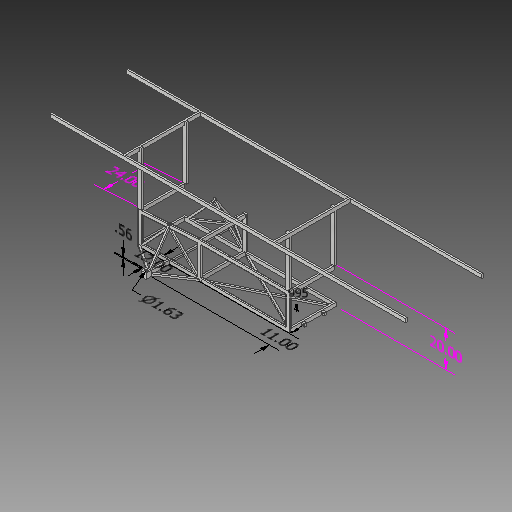
# Autodesk Inventor part: finalDoneskies
Saved by Autodesk Inventor 2018 (Build 220112000, 112)
## iProperties
Created: 2018-01-31
Part Number: finalDoneskies
Material: Generic
Document SubType Name: Modeling
Designer: rochee19
Density: 1 g/cm^3
Appearance: Default
Author: rochee19
Autodesk Inventor part; units mm, degrees
ref_plane "YZ Plane" through (0, 0, 0) normal (1, 0, 0) x (0, 1, 0)
ref_plane "XZ Plane" through (0, 0, 0) normal (0, 1, 0) x (-1, 0, 0)
ref_plane "XY Plane" through (0, 0, 0) normal (0, 0, 1) x (1, 0, 0)
sketch "Sketch1" plane through (0, 0, 0) normal (0, 0, 1) x (1, 0, 0)
  line L0 (0, 0) -> (2133.6, 0)
  line L1 (2133.6, 0) -> (2133.6, -50.8)
  line L2 (2133.6, -50.8) -> (0, -50.8)
  line L3 (0, -50.8) -> (0, 0)
  line L4 (2133.6, 0) -> (2082.8, 0)
  line L5 (2082.8, 0) -> (2082.8, 457.2)
  line L6 (2082.8, 457.2) -> (2133.6, 457.2)
  line L7 (2133.6, 457.2) -> (2133.6, 0)
  line L8 (0, 0) -> (50.8, 0)
  line L9 (50.8, 0) -> (50.8, 406.4)
  line L10 (50.8, 406.4) -> (0, 406.4)
  line L11 (0, 406.4) -> (0, 0)
  line L12 (50.8, 203.2) -> (838.2, 203.2)
  line L13 (838.2, 0) -> (889, 0)
  line L14 (889, 0) -> (889, 457.2)
  line L15 (889, 457.2) -> (838.2, 457.2)
  line L16 (838.2, 457.2) -> (838.2, 0)
  dimension "d0" = 2133.6
  dimension "d1" = 50.8
  dimension "d2" = 50.8
  dimension "d3" = 457.2
  dimension "d4" = 50.8
  dimension "d5" = 406.4
  dimension "d6" = 787.4
  dimension "d7" = 50.8
  dimension "d8" = 457.2
  constraints: 34 end point, 8 parallel, 5 horizontal, 4 perpendicular, 1 midpoint, 1 point on line
  measures "d0" distance of L1.end L2.end
  measures "d1" distance of L0.end L1.end
  measures "d2" distance of L5.end L6.end
  measures "d3" distance of L4.end L5.end
  measures "d4" distance of L10.end L9.end
  measures "d5" distance of L9.end L8.end
  measures "d6" distance of L12.start L12.end
  measures "d7" distance of L15.end L14.end
  measures "d8" distance of L14.end L13.end
extrude "Extrusion1" add sketch "Sketch1" along normal blind 25.4 contours L11 L10 L9 L0 | L16 L15 L14 L0 | L0 L5 L6 L7
sketch "Sketch2" plane through (0, 0, 25.4) normal (0, 0, 1) x (1, 0, 0)
  line L0 (0, 0) -> (50.8, 0) projected
  line L1 (0, 0) -> (2133.6, 0)
  line L2 (2133.6, 0) -> (2133.6, -50.8)
  line L3 (2133.6, -50.8) -> (0, -50.8)
  line L4 (0, -50.8) -> (0, 0)
  dimension "d11" = 2133.6
  dimension "d12" = 50.8
  constraints: 8 end point, 2 parallel, 1 horizontal, 1 perpendicular
  measures "d11" distance of L2.end L3.end
  measures "d12" distance of L1.end L2.end
extrude "Extrusion2" add sketch "Sketch2" against normal blind 25.4
sketch "Sketch3" plane through (0, 0, 25.4) normal (0, 0, 1) x (1, 0, 0)
  line L0 (838.2, 457.2) -> (838.2, 0) projected
  line L1 (50.8, 406.4) -> (0, 406.4) projected
  line L2 (838.2, 457.2) -> (25.4, 406.4)
  line L3 (25.4, 406.4) -> (28.5688, 355.6989)
  line L4 (28.5688, 355.6989) -> (841.3688, 406.4989)
  line L5 (841.3688, 406.4989) -> (838.2, 457.2)
  line L6 (889, 0) -> (889, 457.2) projected
  line L7 (2082.8, 457.2) -> (2082.8, 0) projected
  line L8 (889, 457.2) -> (2082.8, 457.2)
  line L9 (2082.8, 457.2) -> (2082.8, 406.4)
  line L10 (2082.8, 406.4) -> (889, 406.4)
  line L11 (889, 406.4) -> (889, 457.2)
  point P0 (0, 0)
  dimension "d15" = 50.8
  constraints: 16 end point, 4 parallel, 3 perpendicular, 1 midpoint
  measures "d15" distance of L3.end L2.end
extrude "Extrusion3" add sketch "Sketch3" against normal blind 25.4
shell "Shell1" thickness 2.54 removed faces 0
sketch "Sketch5" plane through (0, 0, 0) normal (0, 0, -1) x (-1, 0, 0)
  line L0 (-2133.6, -50.8) -> (0, -50.8) projected
  line L1 (0, -50.8) -> (-25.4, -50.8)
  line L2 (-25.4, -50.8) -> (-25.4, 0)
  line L3 (-25.4, 0) -> (0, 0)
  line L4 (0, 0) -> (0, -50.8)
  line L5 (-2133.6, 457.2) -> (-2133.6, -50.8) projected
  line L6 (-2133.6, -50.8) -> (-2108.2, -50.8)
  line L7 (-2108.2, -50.8) -> (-2108.2, 0)
  line L8 (-2108.2, 0) -> (-2133.6, 0)
  line L9 (-2133.6, 0) -> (-2133.6, -50.8)
  line L10 (-2082.8, 406.4) -> (-889, 0) projected
  line L11 (-889, 0) -> (-889, -50.8)
  line L12 (-838.2, 406.3009) -> (-838.2, 0) projected
  line L13 (-838.2, 0) -> (-838.2, -50.8)
  line L14 (-838.2, -25.4) -> (-889, -25.4)
  line L15 (-876.3, -50.8) -> (-850.9, -50.8)
  line L16 (-850.9, -50.8) -> (-850.9, 0)
  line L17 (-850.9, 0) -> (-876.3, 0)
  line L18 (-876.3, 0) -> (-876.3, -50.8)
  line L19 (-876.3, -50.8) -> (-850.9, 0) construction
  line L20 (-850.9, -50.8) -> (-876.3, 0) construction
  line L21 (-838.2, -25.4) -> (-25.4, -25.4)
  line L22 (-431.8, -25.4) -> (-431.8, 0)
  line L23 (-48.26, -2.54) -> (-840.74, -2.54) projected
  line L24 (-431.8, 0) -> (-431.8, -50.8)
  line L25 (-50.8, 0) -> (-838.2, 0) projected
  line L26 (-444.5, -50.8) -> (-419.1, -50.8)
  line L27 (-419.1, -50.8) -> (-419.1, 0)
  line L28 (-419.1, 0) -> (-444.5, 0)
  line L29 (-444.5, 0) -> (-444.5, -50.8)
  line L30 (-444.5, -50.8) -> (-419.1, 0) construction
  line L31 (-419.1, -50.8) -> (-444.5, 0) construction
  point P0 (-863.6, -25.4)
  point P1 (-788.4519, -2.54)
  point P2 (-776.7012, 0)
  dimension "d23" = 25.4
  dimension "d24" = 50.8
  dimension "d25" = 25.4
  dimension "d26" = 25.4
  dimension "d27" = 50.8
  dimension "d28" = 25.4
  constraints: 52 end point, 9 midpoint, 8 parallel, 7 perpendicular, 6 point on line, 4 horizontal
  measures "d23" distance of L2.end L3.end
  measures "d24" distance of L1.end L2.end
  measures "d25" distance of L8.end L7.end
  measures "d26" distance of L17.end L16.end
  measures "d27" distance of L16.end L15.end
  measures "d28" distance of L28.end L27.end
extrude "Extrusion5" add sketch "Sketch5" along normal blind 609.6 contours L5 L8 L7 L0 | L18 L14 L16 L0 | L18 L17 L16 L14 | L29 L21 L24 L0 | L24 L21 L27 L0 | L29 L23 L22 L21 | L22 L23 L27 L21 | L29 L25 L22 L23 | L2 L3 L4 L0 | L22 L25 L27 L23
sketch "Sketch6" plane through (0, 0, -609.6) normal (0, 0, -1) x (-1, 0, 0)
  line L0 (-2133.6, 457.2) -> (-2133.6, -50.8) projected
  line L1 (-2133.6, -50.8) -> (0, -50.8)
  line L2 (0, -50.8) -> (0, 0)
  line L3 (0, 0) -> (-2133.6, 0)
  line L4 (-2133.6, 0) -> (-2133.6, -50.8)
  constraints: 8 end point, 2 parallel, 1 horizontal, 1 perpendicular
extrude "Extrusion6" add sketch "Sketch6" along normal blind 25.4
sketch "Sketch7" plane through (0, 0, -635) normal (0, 0, -1) x (-1, 0, 0)
  line L0 (-889, 0) -> (-838.2, 0)
  line L1 (-838.2, 0) -> (-838.2, 457.2)
  line L2 (-838.2, 457.2) -> (-889, 457.2)
  line L3 (-889, 457.2) -> (-889, 0)
  line L4 (0, 406.4) -> (0, -50.8) projected
  line L5 (0, 406.4) -> (-50.8, 406.4)
  line L6 (-50.8, 406.4) -> (-50.8, 0)
  line L7 (-50.8, 0) -> (0, 0)
  line L8 (0, 0) -> (0, 406.4)
  line L9 (-2133.6, 0) -> (-2133.6, -50.8) projected
  line L10 (-2133.6, 0) -> (-2082.8, 0)
  line L11 (-2082.8, 0) -> (-2082.8, 457.2)
  line L12 (-2082.8, 457.2) -> (-2133.6, 457.2)
  line L13 (-2133.6, 457.2) -> (-2133.6, 0)
  line L14 (-2082.8, 406.4) -> (-889, 406.4)
  line L15 (-889, 406.4) -> (-889, 457.2)
  line L16 (-889, 457.2) -> (-2082.8, 457.2)
  line L17 (-2082.8, 457.2) -> (-2082.8, 406.4)
  line L18 (-25.4, 406.4) -> (0, 406.4) projected
  line L19 (-838.2, 457.2) -> (-25.4, 406.4)
  line L20 (-25.4, 406.4) -> (-28.5688, 355.6989)
  line L21 (-28.5688, 355.6989) -> (-841.3688, 406.4989)
  line L22 (-841.3688, 406.4989) -> (-838.2, 457.2)
  line L23 (-838.2, 406.3009) -> (-50.8, 357.0884) projected
  line L24 (-50.8, 357.0884) -> (-838.2, 0) projected
  line L25 (-50.8, 357.0884) -> (-838.2, 0)
  line L26 (-838.2, 0) -> (-827.7094, -23.1324)
  line L27 (-827.7094, -23.1324) -> (-40.3094, 333.956)
  line L28 (-40.3094, 333.956) -> (-50.8, 357.0884)
  line L29 (-2082.8, 406.4) -> (-889, 406.4) projected
  dimension "d33" = 50.8
  dimension "d34" = 457.2
  dimension "d35" = 50.8
  dimension "d36" = 457.2
  dimension "d37" = 50.8
  dimension "d38" = 25.4
  constraints: 48 end point, 13 equal length, 6 perpendicular, 4 horizontal
  measures "d33" distance of L2.end L1.end
  measures "d34" distance of L1.end L0.end
  measures "d35" distance of L12.end L11.end
  measures "d36" distance of L11.end L10.end
  measures "d37" distance of L18.start L20.end
  measures "d38" distance of L26.end L0.end
extrude "Extrusion7" [suppressed]
sketch "Sketch8" plane through (0, 0, -635) normal (0, 0, -1) x (-1, 0, 0)
  line L0 (0, 0) -> (-2133.6, 0) projected
  line L1 (-889, 0) -> (-838.2, 0)
  line L2 (-838.2, 0) -> (-838.2, 457.2)
  line L3 (-838.2, 457.2) -> (-889, 457.2)
  line L4 (-889, 457.2) -> (-889, 0)
  dimension "d42" = 50.8
  dimension "d43" = 457.2
  constraints: 8 end point, 2 parallel, 1 horizontal, 1 perpendicular
  measures "d42" distance of L3.end L2.end
  measures "d43" distance of L2.end L1.end
extrude "Extrusion8" add sketch "Sketch8" against normal blind 25.4
sketch "Sketch9" plane through (0, 0, 0) normal (0, 0, -1) x (-1, 0, 0)
  line L0 (0, 406.4) -> (0, 0) projected
  line L1 (0, 406.4) -> (-25.4, 406.4)
  line L2 (-25.4, 406.4) -> (-25.4, 355.6)
  line L3 (-25.4, 355.6) -> (0, 355.6)
  line L4 (0, 355.6) -> (0, 406.4)
  dimension "d46" = 25.4
  dimension "d47" = 50.8
  constraints: 8 end point, 2 parallel, 1 horizontal, 1 perpendicular
  measures "d46" distance of L3.end L2.end
  measures "d47" distance of L2.end L1.end
sketch "Sketch10" plane through (0, 0, -635) normal (0, 0, -1) x (-1, 0, 0)
  line L0 (-889, 457.2) -> (-889, 0) projected
  line L1 (-50.8, 357.0884) -> (-838.2, 406.3009) projected
  line L2 (-889, 406.4) -> (-838.2, 406.3009)
  line L3 (-838.2, 406.3009) -> (-863.6, 406.3504)
  line L4 (-889, 457.2) -> (-838.2, 457.2) projected
  line L5 (-863.6, 457.2) -> (-863.6, 406.3504)
  line L6 (-876.3, 406.3752) -> (-850.9, 406.3752)
  line L7 (-850.9, 406.3752) -> (-850.9, 457.1752)
  line L8 (-850.9, 457.1752) -> (-876.3, 457.1752)
  line L9 (-876.3, 457.1752) -> (-876.3, 406.3752)
  line L10 (-876.3, 406.3752) -> (-850.9, 457.1752) construction
  line L11 (-850.9, 406.3752) -> (-876.3, 457.1752) construction
  point P0 (0, 0)
  point P1 (-2133.6, 457.2)
  point P2 (-863.6, 431.7752)
  dimension "d48" = 25.4
  dimension "d49" = 50.8
  constraints: 18 end point, 5 midpoint, 2 parallel, 2 perpendicular, 1 horizontal
  measures "d48" distance of L8.end L7.end
  measures "d49" distance of L7.end L6.end
extrude "Extrusion9" add sketch "Sketch10" against normal blind 635 contours L9 L8 L5 L6 | L8 L7 L6 L5
extrude "Extrusion10" add sketch "Sketch9" along normal blind 609.6
sketch "Sketch11" plane through (0, 0, 0) normal (0, 0, -1) x (-1, 0, 0)
  line L0 (-889, 457.2) -> (-838.2, 457.2) projected
  line L1 (-2133.6, 457.2) -> (-2108.2, 457.2)
  line L2 (-2108.2, 457.2) -> (-2108.2, 406.4)
  line L3 (-2108.2, 406.4) -> (-2133.6, 406.4)
  line L4 (-2133.6, 406.4) -> (-2133.6, 457.2)
  point P0 (0, 0)
  dimension "d54" = 25.4
  dimension "d55" = 50.8
  constraints: 8 end point, 2 parallel, 1 horizontal, 1 perpendicular
  measures "d54" distance of L2.end L3.end
  measures "d55" distance of L1.end L2.end
extrude "Extrusion11" add sketch "Sketch11" along normal blind 609.6
sketch "Sketch12" plane through (2133.6, -50.8, 25.4) normal (1, 0, 0) x (0, 0, -1)
  line L0 (635, 0) -> (635, 50.8) projected
  line L1 (635, 50.8) -> (635, 0)
  line L2 (635, 25.4) -> (0, 25.4)
  line L3 (0, 508) -> (0, 0) projected
  line L4 (25.4, 50.8) -> (0, 50.8) projected
  line L5 (25.4, 50.8) -> (25.4, 0)
  line L6 (22.86, 2.54) -> (22.86, 505.46) projected
  line L7 (25.4, 50.8) -> (25.4, 0) projected
  line L8 (25.4, 25.4) -> (635, 25.4)
  line L9 (330.2, 25.4) -> (330.2, 50.8)
  line L10 (25.4, 50.8) -> (635, 50.8) projected
  line L11 (330.2, 25.4) -> (209.55, 25.4)
  line L12 (209.55, 25.4) -> (450.85, 25.4)
  line L13 (450.85, 25.4) -> (482.6, 25.4)
  line L14 (450.85, 6.35) -> (450.85, 44.45)
  line L15 (450.85, 44.45) -> (482.6, 44.45)
  line L16 (482.6, 44.45) -> (482.6, 6.35)
  line L17 (482.6, 6.35) -> (450.85, 6.35)
  line L18 (450.85, 6.35) -> (482.6, 44.45) construction
  line L19 (450.85, 44.45) -> (482.6, 6.35) construction
  line L20 (209.55, 25.4) -> (177.8, 25.4)
  line L21 (177.8, 25.4) -> (209.55, 25.4)
  line L22 (177.8, 6.35) -> (177.8, 44.45)
  line L23 (177.8, 44.45) -> (209.55, 44.45)
  line L24 (209.55, 44.45) -> (209.55, 6.35)
  line L25 (209.55, 6.35) -> (177.8, 6.35)
  line L26 (177.8, 6.35) -> (209.55, 44.45) construction
  line L27 (177.8, 44.45) -> (209.55, 6.35) construction
  point P0 (466.725, 25.4)
  point P1 (193.675, 25.4)
  dimension "d58" = 120.65
  dimension "d59" = 241.3
  dimension "d60" = 31.75
  dimension "d61" = 38.1
  dimension "d62" = 31.75
  dimension "d63" = 38.1
  constraints: 44 end point, 10 midpoint, 5 parallel, 5 point on line, 4 perpendicular, 2 collinear, 1 horizontal, 1 vertical
  measures "d58" distance of L9.start L11.end
  measures "d59" distance of L11.end L12.end
  measures "d60" distance of L12.end L13.end
  measures "d61" distance of L14.start L14.end
  measures "d62" distance of L11.end L20.end
  measures "d63" distance of L22.start L22.end
extrude "Extrusion12" add sketch "Sketch12" along normal blind 38.1 contours L16 L17 L14 L2 | L2 L14 L15 L16 | L24 L25 L22 L2 | L2 L22 L23 L24
sketch "Sketch13" plane through (2133.6, -44.45, -152.4) normal (0, 0, 1) x (1, 0, 0)
  line L0 (0, 38.1) -> (38.1, 38.1) projected
  line L1 (19.05, 38.1) -> (19.05, 0)
  line L2 (0, 0) -> (38.1, 0) projected
  circle A0 centre (19.05, 19.05) radius 8.128
  point P0 (-2133.6, 44.45)
  dimension "d66" = 16.256
  constraints: 3 midpoint, 2 end point, 1 centre point
  measures "d66" diameter of A0
extrude "Extrusion13" cut sketch "Sketch13" against normal blind 38.1
sketch "Sketch14" plane through (2133.6, -44.45, -457.2) normal (0, 0, -1) x (-1, 0, 0)
  line L0 (0, 38.1) -> (-38.1, 38.1) projected
  line L1 (-19.05, 38.1) -> (-19.05, 0)
  line L2 (0, 0) -> (-38.1, 0) projected
  circle A0 centre (-19.05, 19.05) radius 8.128
  point P0 (2133.6, 44.45)
  constraints: 3 midpoint, 2 end point, 1 centre point
extrude "Extrusion14" cut sketch "Sketch14" against normal blind 38.1
sketch "Sketch23" plane through (0, 0, 25.4) normal (0, 0, 1) x (1, 0, 0)
  line L0 (50.8, 0) -> (50.8, 357.0884) projected
  line L1 (50.8, 0) -> (50.8, -50.8)
  line L2 (2133.6, -50.8) -> (0, -50.8) projected
  line L3 (50.8, 357.0884) -> (838.2, 0) projected
  line L4 (838.2, 0) -> (838.2, -50.8)
  line L5 (838.2, -50.8) -> (838.2, -25.4)
  line L6 (838.2, -25.4) -> (50.8, -25.4)
  line L7 (419.1, 0) -> (419.1, -50.8) projected
  line L8 (419.1, -25.4) -> (419.1, 0)
  line L9 (419.1, 0) -> (419.1, -50.8)
  line L10 (419.1, 0) -> (444.5, 0)
  line L11 (50.8, 0) -> (2082.8, 0) projected
  line L12 (444.5, -50.8) -> (444.5, 0) projected
  line L13 (444.5, -50.8) -> (444.5, 0)
  line L14 (444.5, 0) -> (444.5, -25.4)
  line L15 (419.1, -50.8) -> (444.5, -50.8)
  line L16 (444.5, -50.8) -> (444.5, 0)
  line L17 (444.5, 0) -> (419.1, 0)
  line L18 (419.1, 0) -> (419.1, -50.8)
  line L19 (419.1, -50.8) -> (444.5, 0) construction
  line L20 (444.5, -50.8) -> (419.1, 0) construction
  point P0 (0, 0)
  point P1 (50.8, 329.1985)
  point P2 (776.7012, 0)
  point P3 (431.8, -25.4)
  constraints: 30 end point, 6 midpoint, 3 collinear, 3 point on line, 2 parallel, 2 vertical, 1 horizontal, 1 perpendicular
extrude "Extrusion20" add sketch "Sketch23" along normal blind 279.4 contours L10 L12 L6 L7 | L6 L12 L2 L7
sketch "Sketch24" plane through (0, 0, -635) normal (0, 0, -1) x (-1, 0, 0)
  line L0 (-444.5, 0) -> (-444.5, -50.8)
  line L1 (-444.5, -50.8) -> (-419.1, -50.8)
  line L2 (-419.1, -50.8) -> (-419.1, 0)
  line L3 (-419.1, 0) -> (-444.5, 0)
  line L4 (0, 0) -> (-838.2, 0) projected
  point P0 (-50.8, 0)
  point P1 (-776.7012, 0)
  constraints: 8 end point, 2 perpendicular, 1 collinear, 1 vertical
extrude "Extrusion21" add sketch "Sketch24" along normal blind 279.4
sketch "Sketch25" plane through (2133.6, -50.8, -635) normal (0, -1, 0) x (1, 0, 0)
  line L0 (-2133.6, 660.4) -> (-2133.6, 0) projected
  line L1 (-1714.5, 660.4) -> (-1714.5, 939.8) projected
  line L2 (-2133.6, 660.4) -> (-1714.5, 939.8)
  line L3 (-1714.5, 939.8) -> (-1700.4106, 918.6659)
  line L4 (-1700.4106, 918.6659) -> (-2119.5106, 639.2659)
  line L5 (-2119.5106, 639.2659) -> (-2133.6, 660.4)
  line L6 (-1714.5, 939.8) -> (-2133.6, 660.4)
  line L7 (-1714.5, 939.8) -> (-1689.1, 939.8) projected
  line L8 (-1689.1, 939.8) -> (-1269.9857, 660.4)
  line L9 (0, 660.4) -> (-1295.4, 660.4) projected
  line L10 (-1269.9857, 660.4) -> (-1286.2971, 635.9321)
  line L11 (-1286.2971, 635.9321) -> (-1705.4114, 915.3321)
  line L12 (-1705.4114, 915.3321) -> (-1689.1, 939.8)
  point P0 (-2133.6, 635)
  dimension "d102" = 25.4
  dimension "d103" = 503.7074
  dimension "d104" = 503.7074
  constraints: 18 end point, 3 equal length, 3 perpendicular, 2 point on line
  measures "d102" distance of L1.end L3.end
  measures "d103" distance of L7.end L8.end
  measures "d104" distance of L10.end L11.end
extrude "Extrusion22" add sketch "Sketch25" against normal blind 25.4
sketch "Sketch26" plane through (2133.6, -50.8, -635) normal (0, -1, 0) x (1, 0, 0)
  line L0 (-1714.5, 0) -> (-1714.5, -279.4) projected
  line L1 (-2133.6, 25.4) -> (-2133.6, 660.4) projected
  line L2 (-1714.5, -279.4) -> (-2133.6, 0)
  line L3 (-2133.6, 0) -> (-2119.5106, 21.1341)
  line L4 (-2119.5106, 21.1341) -> (-1700.4106, -258.2659)
  line L5 (-1700.4106, -258.2659) -> (-1714.5, -279.4)
  line L6 (-1689.1, 0) -> (-1689.1, -279.4) projected
  line L7 (-1689.1, -279.4) -> (-1266.2023, -5.7603)
  line L8 (-1266.2023, -5.7603) -> (-1280.0009, 15.5648)
  line L9 (-1280.0009, 15.5648) -> (-1702.8986, -258.0749)
  line L10 (-1702.8986, -258.0749) -> (-1689.1, -279.4)
  point P0 (-2133.6, 635)
  dimension "d107" = 25.4
  dimension "d108" = 503.7074
  dimension "d109" = 25.4
  constraints: 16 end point, 4 parallel, 2 perpendicular
  measures "d107" distance of L2.end L3.end
  measures "d108" distance of L6.end L7.end
  measures "d109" distance of L8.end L7.end
extrude "Extrusion23" add sketch "Sketch26" against normal blind 25.4
sketch "Sketch28" plane through (419.1, -50.8, -635) normal (-1, 0, 0) x (0, 0, 1)
  line L0 (879.0384, 50.8) -> (617.9284, 448.692) projected
  line L1 (42.4716, 448.692) -> (-218.6384, 50.8) projected
  line L2 (617.9284, 448.692) -> (42.4716, 448.692)
  line L3 (42.4716, 448.692) -> (42.4716, 499.492)
  line L4 (42.4716, 499.492) -> (617.9284, 499.492)
  line L5 (617.9284, 499.492) -> (617.9284, 448.692)
  line L6 (-279.4, 50.8) -> (0, 476.5632) projected
  line L7 (42.4716, 499.492) -> (0, 476.5632)
  line L8 (0, 476.5632) -> (24.1328, 431.8614)
  line L9 (24.1328, 431.8614) -> (66.6043, 454.7902)
  line L10 (66.6043, 454.7902) -> (42.4716, 499.492)
  line L11 (660.4, 50.8) -> (660.4, 0) projected
  line L12 (617.9284, 499.492) -> (660.4, 476.5632)
  line L13 (660.4, 476.5632) -> (636.2672, 431.8614)
  line L14 (636.2672, 431.8614) -> (593.7957, 454.7902)
  line L15 (593.7957, 454.7902) -> (617.9284, 499.492)
  point P0 (635, 50.8)
  point P1 (660.4, 432.4946)
  dimension "d116" = 50.8
  dimension "d117" = 50.8
  dimension "d118" = 50.8
  constraints: 24 end point, 6 parallel, 3 perpendicular, 1 horizontal
  measures "d116" distance of L1.start L3.end
  measures "d117" distance of L8.end L6.end
  measures "d118" distance of L12.end L13.end
extrude "Extrusion25" add sketch "Sketch28" against normal blind 25.4
sketch "Sketch29" plane through (2133.6, -50.8, -635) normal (0, -1, 0) x (1, 0, 0)
  line L0 (-1257.3, 25.4) -> (-1257.3, 635) projected
  line L1 (-25.4, 635) -> (-1295.4, 635) projected
  line L2 (-1257.3, 25.4) -> (-25.4, 635)
  line L3 (-25.4, 635) -> (-14.1347, 612.2348)
  line L4 (-14.1347, 612.2348) -> (-1246.0347, 2.6348)
  line L5 (-1246.0347, 2.6348) -> (-1257.3, 25.4)
  line L6 (-1257.3, 635) -> (-1282.7, 635) projected
  line L7 (-1257.3, 635) -> (-25.4, 25.4)
  line L8 (-25.4, 25.4) -> (-14.1347, 48.1652)
  line L9 (-14.1347, 48.1652) -> (-1246.0347, 657.7652)
  line L10 (-1246.0347, 657.7652) -> (-1257.3, 635)
  point P0 (-2133.6, 635)
  dimension "d121" = 25.4
  dimension "d122" = 25.4
  constraints: 16 end point, 4 parallel, 2 perpendicular
  measures "d121" distance of L1.start L3.end
  measures "d122" distance of L8.end L7.end
extrude "Extrusion26" add sketch "Sketch29" against normal blind 25.4 contours L2 L7 L4 L5 | L10 L9 L1 | L1 L9 L2 L7 | L2 L9 L4 L7 | L2 L3 L4 L9 | L4 L9 L8 L7
extrude "Extrusion28" [suppressed]
sketch "Sketch33" plane through (0, -12.7, -596.9) normal (0, 0, 1) x (1, 0, 0)
  line L0 (-152.4, 0) -> (-152.4, 12.7) projected
  line L1 (0, 12.7) -> (-152.4, 12.7) projected
  line L2 (-152.4, 0) -> (-139.7, 0)
  line L3 (-139.7, 0) -> (-139.7, 12.7)
  line L4 (-139.7, 12.7) -> (-152.4, 12.7)
  line L5 (-152.4, 12.7) -> (-152.4, 0)
  line L6 (-152.4, 368.3) -> (-152.4, 381) projected
  line L7 (0, 368.3) -> (-152.4, 368.3) projected
  line L8 (-152.4, 381) -> (-139.7, 381)
  line L9 (-139.7, 381) -> (-139.7, 368.3)
  line L10 (-139.7, 368.3) -> (-152.4, 368.3)
  line L11 (-152.4, 368.3) -> (-152.4, 381)
  dimension "d139" = 12.7
  dimension "d140" = 12.7
  constraints: 16 end point, 4 parallel, 2 horizontal, 2 perpendicular, 2 point on line
  measures "d139" distance of L4.end L3.end
  measures "d140" distance of L9.end L10.end
extrude "Extrusion29" [suppressed]
sketch "Sketch51" plane through (444.5, -50.8, -635) normal (1, 0, 0) x (0, 0, -1)
  line L0 (-939.8, 25.4) -> (-939.8, 50.8) projected
  line L1 (-617.9284, 499.492) -> (-647.7476, 483.3937) projected
  line L2 (-939.8, 50.8) -> (-647.7476, 483.3937)
  line L3 (-647.7476, 483.3937) -> (-626.696, 469.1814)
  line L4 (-626.696, 469.1814) -> (-918.7484, 36.5877)
  line L5 (-918.7484, 36.5877) -> (-939.8, 50.8)
  line L6 (279.4, 50.8) -> (279.4, 25.4) projected
  line L7 (0, 476.5632) -> (-42.4716, 499.492) projected
  line L8 (279.4, 50.8) -> (-12.6524, 483.3937)
  line L9 (-12.6524, 483.3937) -> (-33.704, 469.1814)
  line L10 (-33.704, 469.1814) -> (258.3484, 36.5877)
  line L11 (258.3484, 36.5877) -> (279.4, 50.8)
  point P0 (-635, 50.8)
  dimension "d223" = 25.4
  dimension "d224" = 25.4
  constraints: 16 end point, 4 parallel, 2 perpendicular
  measures "d223" distance of L1.end L3.end
  measures "d224" distance of L9.end L8.end
extrude "Extrusion44" add sketch "Sketch51" against normal blind 25.4
sketch "Sketch74" plane through (0, 0, -635) normal (0, 0, -1) x (-1, 0, 0)
  line L0 (-2133.6, 457.2) -> (-2133.6, 406.4) projected
  line L1 (-2133.6, 406.4) -> (-2133.6, 457.2)
  line L2 (-2133.6, 457.2) -> (-2146.3, 457.2) projected
  line L3 (-2133.6, 457.2) -> (-2082.8, 457.2)
  line L4 (-2082.8, 457.2) -> (-2082.8, 1168.4)
  line L5 (-2082.8, 1168.4) -> (-2133.6, 1168.4)
  line L6 (-2133.6, 1168.4) -> (-2133.6, 457.2)
  line L7 (0, -25.4) -> (0, 0) projected
  line L8 (0, 406.4) -> (-50.8, 406.4)
  line L9 (-50.8, 406.4) -> (-50.8, 1168.4)
  line L10 (-50.8, 1168.4) -> (0, 1168.4)
  line L11 (0, 1168.4) -> (0, 406.4)
  dimension "d275" = 50.8
  dimension "d276" = 711.2
  dimension "d277" = 50.8
  constraints: 18 end point, 5 equal length, 2 horizontal, 2 perpendicular, 1 point on line
  measures "d275" distance of L5.end L4.end
  measures "d276" distance of L4.end L3.end
  measures "d277" distance of L9.end L10.end
extrude "Extrusion62" add sketch "Sketch74" against normal blind 25.4
sketch "Sketch75" plane through (0, 0, 25.4) normal (0, 0, 1) x (1, 0, 0)
  line L0 (0, 406.4) -> (0, -25.4) projected
  line L1 (0, 406.4) -> (50.8, 406.4)
  line L2 (50.8, 406.4) -> (50.8, 1168.4)
  line L3 (50.8, 1168.4) -> (0, 1168.4)
  line L4 (0, 1168.4) -> (0, 406.4)
  line L5 (838.2, 457.2) -> (889, 457.2) projected
  line L6 (2133.6, 1168.4) -> (2082.8, 1168.4) projected
  line L7 (2133.6, 457.2) -> (2082.8, 457.2)
  line L8 (2082.8, 457.2) -> (2082.8, 1168.4)
  line L9 (2082.8, 1168.4) -> (2133.6, 1168.4)
  line L10 (2133.6, 1168.4) -> (2133.6, 457.2)
  point P0 (0, 0)
  point P1 (2139.95, 457.2)
  constraints: 16 end point, 4 parallel, 2 horizontal, 2 perpendicular
extrude "Extrusion63" add sketch "Sketch75" against normal blind 25.4
sketch "Sketch79" plane through (2133.6, -50.8, 25.4) normal (1, 0, 0) x (0, 0, -1)
  line L0 (25.4, 407.8884) -> (25.4, 50.8) projected
  point P0 (635, 1193.8)
extrude "Extrusion66" [suppressed]
sketch "Sketch80" plane through (0, 0, 25.4) normal (0, 0, 1) x (1, 0, 0)
  line L0 (48.26, -2.54) -> (48.26, 359.4746) projected
  line L1 (444.5, 397.892) -> (419.1, 397.892) projected
  line L2 (48.26, -2.54) -> (419.1, 397.892)
  line L3 (419.1, 397.892) -> (437.7359, 380.6333)
  line L4 (437.7359, 380.6333) -> (66.8959, -19.7987)
  line L5 (66.8959, -19.7987) -> (48.26, -2.54)
  line L6 (838.2, 406.3009) -> (838.2, 0) projected
  line L7 (838.2, 0) -> (443.4121, 397.892)
  line L8 (443.4121, 397.892) -> (425.3814, 380.0019)
  line L9 (425.3814, 380.0019) -> (820.1693, -17.89)
  line L10 (820.1693, -17.89) -> (838.2, 0)
  point P0 (0, 0)
  dimension "d293" = 25.4
  dimension "d294" = 25.4
  constraints: 16 end point, 4 parallel, 2 perpendicular
  measures "d293" distance of L1.end L3.end
  measures "d294" distance of L8.end L7.end
extrude "Extrusion67" add sketch "Sketch80" against normal blind 25.4 contours L7 L10 L9 L4 L3 L8 | L3 L8 L9 L4 L5 L2 | L3 L4 L9 L8
sketch "Sketch81" plane through (0, 0, 25.4) normal (0, 0, 1) x (1, 0, 0)
  line L0 (2082.8, 406.4) -> (2082.8, 0) projected
  line L1 (889, 0) -> (2082.8, 0) projected
  point P0 (0, 0)
extrude "Extrusion68" [suppressed]
sketch "Sketch82" plane through (0, 0, -635) normal (0, 0, -1) x (-1, 0, 0)
  line L0 (-50.8, 357.0884) -> (-838.2, 0) projected
  line L1 (-50.8, 357.0884) -> (-838.2, 0)
  line L2 (-838.2, 0) -> (-827.7094, -23.1324)
  line L3 (-827.7094, -23.1324) -> (-40.3094, 333.956)
  line L4 (-40.3094, 333.956) -> (-50.8, 357.0884)
  point P0 (0, 0)
  dimension "d300" = 25.4
  constraints: 8 end point, 3 equal length, 1 perpendicular
  measures "d300" distance of L2.end L0.end
extrude "Extrusion69" cut sketch "Sketch82" against normal blind 25.4
sketch "Sketch83" plane through (0, 0, -635) normal (0, 0, -1) x (-1, 0, 0)
  line L0 (-458.6082, 382.5764) -> (-838.2, 0) projected
  line L1 (-444.5, 396.7955) -> (-456.2305, 384.9727) projected
  line L2 (-838.2, 0) -> (-444.5, 396.7955)
  line L3 (-838.2, 0) -> (-444.5, 396.7955)
  line L4 (-444.5, 396.7955) -> (-426.4693, 378.9054)
  line L5 (-426.4693, 378.9054) -> (-820.1693, -17.89)
  line L6 (-820.1693, -17.89) -> (-838.2, 0)
  line L7 (-50.8, 0.2027) -> (-50.8, 357.0884) projected
  line L8 (-50.8, 0.2027) -> (-422.297, 401.1418)
  line L9 (-422.297, 401.1418) -> (-440.9285, 383.8784)
  line L10 (-440.9285, 383.8784) -> (-69.4316, -17.0607)
  line L11 (-69.4316, -17.0607) -> (-50.8, 0.2027)
  point P0 (0, 0)
  dimension "d303" = 25.4
  constraints: 18 end point, 4 parallel, 2 perpendicular, 1 collinear
  measures "d303" distance of L9.end L8.end
extrude "Extrusion70" add sketch "Sketch83" against normal blind 25.4
sketch "Sketch84" plane through (0, 0, -635) normal (0, 0, -1) x (-1, 0, 0)
  line L0 (-838.2, 0) -> (-827.7094, -23.1324) projected
  line L1 (-827.7094, -23.1324) -> (-776.7012, 0) projected
  line L2 (-838.2, 0) -> (-776.7012, 0)
  line L3 (-776.7012, 0) -> (-776.7012, -23.1324)
  line L4 (-776.7012, -23.1324) -> (-838.2, -23.1324)
  line L5 (-838.2, -23.1324) -> (-838.2, 0)
  point P0 (0, 0)
  constraints: 8 end point, 2 parallel, 1 horizontal, 1 perpendicular
extrude "Extrusion71" add sketch "Sketch84" against normal blind 25.4 contours L2 L1 L0
sketch "Sketch85" plane through (0, 406.4, -609.6) normal (-1, 0, 0) x (0, 0, 1)
  line L0 (0, 762) -> (0, 50.8) projected
  line L1 (0, 762) -> (0, 749.3)
  line L2 (609.6, 762) -> (609.6, 736.6)
  line L3 (609.6, 50.8) -> (609.6, 762) projected
  line L4 (609.6, 736.6) -> (0, 736.6)
  line L5 (-245.491, 711.2) -> (855.091, 711.2)
  line L6 (855.091, 711.2) -> (855.091, 762)
  line L7 (855.091, 762) -> (-245.491, 762)
  line L8 (-245.491, 762) -> (-245.491, 711.2)
  line L9 (-245.491, 711.2) -> (855.091, 762) construction
  line L10 (855.091, 711.2) -> (-245.491, 762) construction
  point P0 (609.6, -406.4)
  point P1 (304.8, 736.6)
  dimension "d308" = 12.7
  dimension "d309" = 25.4
  dimension "d310" = 1100.582
  dimension "d311" = 50.8
  constraints: 18 end point, 3 midpoint, 3 point on line, 2 parallel, 2 perpendicular, 1 horizontal
  measures "d308" distance of L0.start L1.end
  measures "d309" distance of L2.start L2.end
  measures "d310" distance of L7.end L6.end
  measures "d311" distance of L6.end L5.end
extrude "Extrusion72" add sketch "Sketch85" against normal blind 25.4
sketch "Sketch86" plane through (2133.6, 457.2, 25.4) normal (1, 0, 0) x (0, 0, -1)
  line L0 (25.4, 711.2) -> (25.4, 0) projected
  line L1 (25.4, 711.2) -> (25.4, 685.8)
  line L2 (25.4, 685.8) -> (635, 685.8)
  line L3 (635, 711.2) -> (635, 0) projected
  line L4 (660.4, 660.4) -> (880.491, 660.4) projected
  line L5 (-220.091, 711.2) -> (880.491, 711.2)
  line L6 (880.491, 711.2) -> (880.491, 660.4)
  line L7 (880.491, 660.4) -> (-220.091, 660.4)
  line L8 (-220.091, 660.4) -> (-220.091, 711.2)
  line L9 (-220.091, 711.2) -> (880.491, 660.4) construction
  line L10 (880.491, 711.2) -> (-220.091, 660.4) construction
  point P0 (25.4, -457.2)
  point P1 (330.2, 685.8)
  dimension "d314" = 25.4
  constraints: 16 end point, 3 midpoint, 2 parallel, 2 perpendicular, 2 point on line, 1 horizontal
  measures "d314" distance of L0.start L1.end
extrude "Extrusion73" add sketch "Sketch86" against normal blind 25.4
sketch "Sketch87" plane through (0, 1117.6, 245.491) normal (0, 0, 1) x (1, 0, 0)
  line L0 (0, 50.8) -> (0, 0) projected
  line L1 (0, 50.8) -> (-1016, 50.8)
  line L2 (-1016, 50.8) -> (3987.8, 50.8)
  line L3 (3987.8, 50.8) -> (3987.8, 0)
  line L4 (3987.8, 0) -> (-1016, 0)
  line L5 (-1016, 0) -> (-1016, 50.8)
  point P0 (0, -1117.6)
  dimension "d317" = 1016
  dimension "d318" = 5003.8
  constraints: 10 end point, 2 horizontal, 2 parallel, 1 perpendicular
  measures "d317" distance of L0.start L1.end
  measures "d318" distance of L3.end L4.end
extrude "Extrusion74" add sketch "Sketch87" against normal blind 25.4
sketch "Sketch88" plane through (0, 1117.6, -855.091) normal (0, 0, -1) x (-1, 0, 0)
  line L0 (1016, 50.8) -> (0, 50.8) projected
  line L1 (-3987.8, 0) -> (-2133.6, 0) projected
  line L2 (1016, 50.8) -> (-3987.8, 50.8)
  line L3 (-3987.8, 50.8) -> (-3987.8, 0)
  line L4 (-3987.8, 0) -> (1016, 0)
  line L5 (1016, 0) -> (1016, 50.8)
  point P0 (0, -1117.6)
  constraints: 8 end point, 2 parallel, 1 horizontal, 1 perpendicular
extrude "Extrusion75" add sketch "Sketch88" against normal blind 25.4
sketch "Sketch95" plane through (0, 0, 304.8) normal (0, 0, 1) x (1, 0, 0)
  line L0 (443.8315, -50.8) -> (419.7685, -50.8) projected
  line L1 (431.8, -50.8) -> (466.725, -50.8)
  line L2 (431.8, -50.8) -> (396.875, -50.8)
  line L3 (419.1, -50.8) -> (444.5, -50.8) projected
  line L4 (396.875, -50.8) -> (396.875, 25.4)
  line L5 (396.875, 25.4) -> (466.725, 25.4)
  line L6 (466.725, 25.4) -> (466.725, -50.8)
  point P0 (0, 0)
  point P1 (71.5448, -50.8)
  dimension "d350" = 34.925
  dimension "d351" = 34.925
  dimension "d352" = 76.2
  constraints: 10 end point, 3 perpendicular, 1 collinear, 1 midpoint, 1 point on line
  measures "d350" distance of L1.start L1.end
  measures "d351" distance of L1.start L2.end
  measures "d352" distance of L2.end L4.end
extrude "Extrusion80" add sketch "Sketch95" along normal blind 69.85
sketch "Sketch96" plane through (396.875, 25.4, 304.8) normal (0, 1, 0) x (1, 0, 0)
  line L0 (69.85, 0) -> (0, 0) projected
  line L1 (34.925, 0) -> (34.925, -69.85)
  line L2 (69.85, -69.85) -> (0, -69.85) projected
  circle A0 centre (34.925, -34.925) radius 15.0812
  point P0 (-396.875, 304.8)
  dimension "d355" = 30.1625
  constraints: 3 midpoint, 2 end point, 1 centre point
  measures "d355" diameter of A0
extrude "Extrusion81" cut sketch "Sketch96" against normal blind 76.2
sketch "Sketch97" plane through (396.875, 25.4, 304.8) normal (0, 1, 0) x (1, 0, 0)
  line L0 (69.85, 0) -> (0, 0) projected
  line L1 (34.925, 0) -> (34.925, -69.85)
  line L2 (0, -69.85) -> (69.85, -69.85) projected
  circle A0 centre (34.925, -34.925) radius 20.6375
  point P0 (-396.875, 304.8)
  dimension "d358" = 41.275
  constraints: 3 midpoint, 2 end point, 1 centre point
  measures "d358" diameter of A0
extrude "Extrusion82" cut sketch "Sketch97" against normal blind 14.2875
sketch "Sketch98" plane through (419.1, 448.692, -17.0716) normal (0, 1, 0) x (1, 0, 0)
  line L0 (0, 608.2166) -> (25.4, 605.2761) projected
  line L1 (25.4, -39.9316) -> (25.4, -19.6116) projected
  line L2 (0, 608.2166) -> (25.4, 608.2166)
  line L3 (25.4, 608.2166) -> (25.4, -32.4529)
  line L4 (25.4, -32.4529) -> (0, -32.4529)
  line L5 (0, -32.4529) -> (0, 608.2166)
  point P0 (-419.1, -17.0716)
  constraints: 8 end point, 2 parallel, 1 horizontal, 1 perpendicular, 1 point on line
extrude "Extrusion83" cut sketch "Sketch98" against normal blind 50.8
sketch "Sketch100" plane through (0, 0, -914.4) normal (0, 0, -1) x (-1, 0, 0)
  line L0 (-466.725, 25.4) -> (-396.875, 25.4) projected
  line L1 (-431.8, 25.4) -> (-396.875, 25.4)
  line L2 (-466.725, -50.8) -> (-466.725, 25.4) projected
  line L3 (-396.875, 25.4) -> (-466.725, 25.4)
  line L4 (-466.725, 25.4) -> (-466.725, -50.8)
  line L5 (-396.875, 25.4) -> (-396.875, -50.8) projected
  line L6 (-466.725, -50.8) -> (-396.875, -50.8)
  line L7 (-396.875, -50.8) -> (-396.875, 25.4)
  point P0 (0, 0)
  constraints: 10 end point, 4 collinear, 1 midpoint, 1 perpendicular
extrude "Extrusion85" add sketch "Sketch100" along normal blind 69.85
sketch "Sketch101" plane through (396.875, 25.4, -914.4) normal (0, 1, 0) x (1, 0, 0)
  line L0 (22.225, 0) -> (47.625, 0) projected
  line L1 (34.925, 0) -> (34.925, 69.85)
  line L2 (69.85, 69.85) -> (0, 69.85) projected
  circle A0 centre (34.925, 34.925) radius 23.8125
  circle A1 centre (34.925, 34.925) radius 10.3188
  point P0 (-396.875, -914.4)
  dimension "d367" = 47.625
  dimension "d368" = 20.6375
  constraints: 3 midpoint, 2 centre point, 2 end point, 1 coincident
  measures "d367" diameter of A0
  measures "d368" diameter of A1
extrude "Extrusion86" cut sketch "Sketch101" against normal blind 127 contours A1 L1 | L1 A1
sketch "Sketch102" plane through (396.875, 25.4, -914.4) normal (0, 1, 0) x (1, 0, 0)
  line L0 (0, 0) -> (69.85, 0) projected
  line L1 (34.925, 0) -> (34.925, 69.6502)
  circle A0 centre (34.925, 34.8251) radius 20.6375
  point P0 (-396.875, -914.4)
  dimension "d371" = 41.275
  constraints: 2 end point, 2 midpoint, 1 centre point, 1 vertical
  measures "d371" diameter of A0
extrude "Extrusion87" cut sketch "Sketch102" against normal blind 14.2875
sketch "Sketch103" plane through (0, -50.8, -635) normal (0, -1, 0) x (1, 0, 0)
  line L0 (396.875, -279.4) -> (396.875, -349.25) projected
  line L1 (396.875, -314.325) -> (466.725, -314.325)
  line L2 (466.725, -279.4) -> (466.725, -349.25) projected
  circle A0 centre (431.8, -314.325) radius 20.6377
  point P0 (0, 635)
  constraints: 3 midpoint, 2 end point, 1 centre point
extrude "Extrusion88" cut sketch "Sketch103" against normal blind 14.2875
sketch "Sketch104" plane through (396.875, 25.4, 304.8) normal (0, 1, 0) x (1, 0, 0)
  point P0 (-396.875, 304.8)
sketch "Sketch105" plane through (419.1, 0, 0) normal (0, 1, 0) x (1, 0, 0)
  line L0 (25.4, 0) -> (25.4, 609.6) projected
  line L1 (25.4, 609.6) -> (0, 609.6)
  line L2 (0, 609.6) -> (0, 0)
  line L3 (0, 0) -> (25.4, 0)
  line L4 (25.4, 0) -> (25.4, 609.6)
  point P0 (-419.1, 0)
  point P1 (25.4, 331.6858)
  dimension "d376" = 25.4
  dimension "d377" = 609.6
  constraints: 8 end point, 2 parallel, 1 horizontal, 1 perpendicular
  measures "d376" distance of L0.start L2.end
  measures "d377" distance of L2.end L1.end
extrude "Extrusion89" cut sketch "Sketch105" against normal blind 25.4
sketch "Sketch118" plane through (838.2, 457.2, 0) normal (0, 1, 0) x (1, 0, 0)
  line L0 (1295.4, -25.4) -> (1270, -25.4) projected
  line L1 (1295.4, -25.4) -> (431.8, -25.4)
  line L2 (431.8, -25.4) -> (431.8, 635)
  line L3 (0, 635) -> (50.8, 635) projected
  line L4 (431.8, 0) -> (431.8, -25.4)
  line L5 (50.8, -25.4) -> (1244.6, -25.4) projected
  line L6 (431.8, -25.4) -> (457.2, -25.4)
  line L7 (457.2, -25.4) -> (457.2, 0)
  line L8 (50.8, 0) -> (1244.6, 0) projected
  circle A0 centre (444.5, -12.7) radius 3.9688
  point P0 (-838.2, 0)
  point P1 (1244.6, 635)
  point P2 (208.4348, -25.4)
  point P3 (208.4348, 0)
  dimension "d423" = 863.6
  dimension "d424" = 25.4
  dimension "d425" = 25.4
  dimension "d426" = 7.9375
  constraints: 10 end point, 4 point on line, 3 perpendicular, 1 centre point, 1 collinear
  measures "d423" distance of L0.start L1.end
  measures "d424" distance of L4.start L1.end
  measures "d425" distance of L1.end L6.end
  measures "d426" diameter of A0
extrude "Extrusion95" cut sketch "Sketch118" against normal blind 76.2 contours A0
sketch "Sketch119" plane through (838.2, 457.2, -635) normal (0, 1, 0) x (1, 0, 0)
  line L0 (1270, 0) -> (1295.4, 0) projected
  line L1 (1295.4, 0) -> (431.8, 0)
  line L2 (0, 0) -> (50.8, 0) projected
  line L3 (431.8, 0) -> (431.8, -25.4)
  line L4 (1244.6, -25.4) -> (50.8, -25.4) projected
  line L5 (431.8, -25.4) -> (457.2, -25.4)
  circle A0 centre (444.5, -12.7) radius 3.9687
  point P0 (-838.2, -635)
  point P1 (1244.6, 0)
  dimension "d429" = 863.6
  dimension "d430" = 25.4
  dimension "d431" = 7.9375
  constraints: 6 end point, 3 point on line, 1 centre point, 1 perpendicular
  measures "d429" distance of L0.end L1.end
  measures "d430" distance of L3.end L5.end
  measures "d431" diameter of A0
extrude "Extrusion96" cut sketch "Sketch119" against normal blind 76.2
sketch "Sketch120" plane through (0, 0, 0) normal (0, 0, -1) x (-1, 0, 0)
  line L0 (-2082.8, 406.4) -> (-889, 406.4) projected
  line L1 (-2082.8, 406.4) -> (-2082.8, 381.1273)
  line L2 (-2085.34, 408.94) -> (-2085.34, -2.54) projected
  point P0 (0, 0)
  point P1 (-2085.34, -2.54)
  dimension "d443" = 25.2727
  constraints: 2 end point, 1 vertical, 1 other
  measures "d443" distance of L0.start L1.end
body "Solid1"
